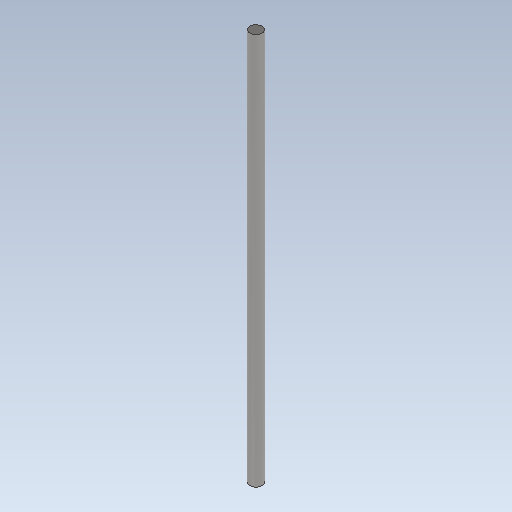
# Autodesk Inventor part: arm shaft
Saved by Autodesk Inventor 2021 (Build 250183000, 183)
## iProperties
Created: 2021-03-29
Part Number: arm shaft
Material: Stainless Steel
Document SubType Name: Modeling
Designer: Work
Mass: 51.4815 g
Surface Area: 41.17 cm^2
Volume: 6.43518 cm^3
Density: 8 g/cm^3
Appearance: Semi-Polished
Author: Work
Autodesk Inventor part; units mm, degrees
ref_plane "YZ Plane" through (0, 0, 0) normal (1, 0, 0) x (0, 1, 0)
ref_plane "XZ Plane" through (0, 0, 0) normal (0, 1, 0) x (-1, 0, 0)
ref_plane "XY Plane" through (0, 0, 0) normal (0, 0, 1) x (1, 0, 0)
sketch "Sketch1" plane through (0, 0, 0) normal (0, 1, 0) x (-1, 0, 0)
  circle A0 centre (0, 0) radius 3.175
  dimension "d0" = 6.35
  constraints: 1 centre point, 1 coincident
  measures "d0" diameter of A0
extrude "Extrusion1" add sketch "Sketch1" along normal blind 203.2
equation "\"d0\" = shaftDiam"
equation "\"d1\" = height"
equation "\"height\" = 203.2"
equation "\"shaftDiam\" = 6.35"
equation "\"stageSpace\" = 2.54"
equation "\"shaftSpace\" = 1.5875"
equation "\"stageAngle\" = 15deg"
equation "\"groundActu\" = 304.8"
equation "\"capThickness\" = 3.175"
equation "\"baseDepth\" = 254"
equation "\"baseWidth\" = 1066.8"
equation "\"stockHeight\" = 50.8"
equation "\"stockWidth\" = 76.2"
equation "\"stockGuage\" = 3.175"
equation "\"stockRad\" = 9.525"
equation "\"sup1Ang\" = 22.619865deg"
equation "\"sup1Len\" = 660.4"
equation "\"supVertLen\" = 955.13561"
equation "\"sup2Ang\" = 8.959949deg"
equation "\"sup2Len\" = 2079.37366"
equation "\"supSideAng\" = 19.376933deg"
equation "\"supSideLen\" = 1531.12879"
equation "\"FlangeDiam\" = 12.7"
equation "\"bearingDiam\" = 9.5504"
equation "\"FlangeDepth\" = 1.5875"
equation "\"smallFilet\" = 0.39687"
equation "\"thickness\" = 12.7"
equation "\"ringDiam\" = 96.46608"
body "Solid1"
